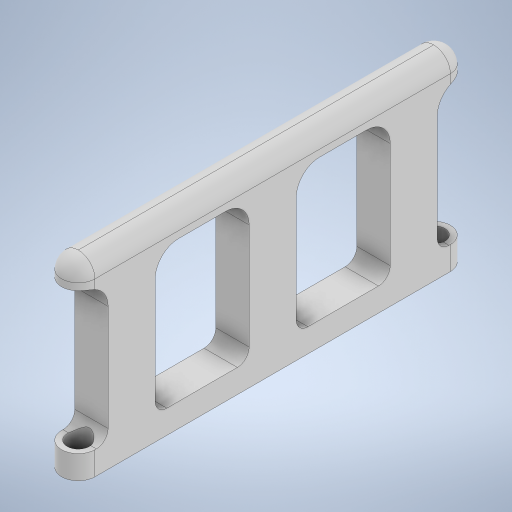
# Autodesk Inventor part: land
Saved by Autodesk Inventor 2023 (Build 270158000, 158)
## iProperties
Created: 2022-11-30
Part Number: land
Material: Generic
Document SubType Name: Modeling
Designer: user
Density: 1 g/cm^3
Appearance: Default
Author: user
Autodesk Inventor part; units mm, degrees
ref_plane "YZ Plane" through (0, 0, 0) normal (1, 0, 0) x (0, 1, 0)
ref_plane "XZ Plane" through (0, 0, 0) normal (0, 1, 0) x (-1, 0, 0)
ref_plane "XY Plane" through (0, 0, 0) normal (0, 0, 1) x (1, 0, 0)
sketch "Sketch1" plane through (0, 0, 0) normal (0, 1, 0) x (-1, 0, 0)
  circle A0 centre (0, 0) radius 4.5
  circle A1 centre (0, 0) radius 1.475
  circle A2 centre (0, 0) radius 3
  line L0 (4.5, 0) -> (4.5, -96.011)
  line L1 (-4.5, 0) -> (-4.5, -96.011)
  circle A3 centre (0, -96.011) radius 4.5
  circle A4 centre (0, -96.011) radius 1.475
  circle A5 centre (0, -96.011) radius 3
  point P0 (2.9871, -99.3766)
  point P1 (-0.7146, -91.5681)
  dimension "d0" = 9
  dimension "d1" = 2.95
  dimension "d2" = 6
  dimension "d3" = 96.011
  dimension "d5" = 9
  dimension "d6" = 2.95
  dimension "d7" = 6
  constraints: 6 centre point, 5 coincident, 4 end point, 4 point on circle, 2 tangent, 2 vertical
  measures "d0" diameter of A0
  measures "d1" diameter of A1
  measures "d2" diameter of A2
  measures "d3" distance of L0.start L0.end
  measures "d5" diameter of A3
  measures "d6" diameter of A4
  measures "d7" diameter of A5
extrude "Extrusion1" add sketch "Sketch1" along normal blind 6.35 contours A0 | L0 A3 L1 A0 | A3 | A1 | A2 | A4 | A5
sketch "Sketch2" plane through (0, 6.35, 0) normal (0, 1, 0) x (1, 0, 0)
  circle A0 centre (0, 0) radius 1.475
  dimension "d10" = 2.95
  constraints: 1 centre point, 1 coincident
  measures "d10" diameter of A0
extrude "Extrusion2" cut sketch "Sketch2" against normal blind 6.35
sketch "Sketch3" plane through (0, 6.35, 0) normal (0, 1, 0) x (1, 0, 0)
  circle A0 centre (0, 0) radius 1.475 projected
  circle A1 centre (0, 0) radius 3
  dimension "d13" = 6
  constraints: 1 centre point, 1 coincident
  measures "d13" diameter of A1
extrude "Extrusion3" cut sketch "Sketch3" against normal blind 5.08
sketch "Sketch4" plane through (0, 6.35, 0) normal (0, 1, 0) x (1, 0, 0)
  arc A0 (4.5, 96.011) -> (-4.5, 96.011) centre (0, 96.011) ccw projected
  circle A1 centre (0, 96.011) radius 1.475
  point P0 (0, 0)
  dimension "d16" = 2.95
  constraints: 1 centre point, 1 coincident
  measures "d16" diameter of A1
extrude "Extrusion4" cut sketch "Sketch4" against normal blind 6.35
sketch "Sketch5" plane through (0, 6.35, 0) normal (0, 1, 0) x (1, 0, 0)
  arc A0 (4.5, 96.011) -> (-4.5, 96.011) centre (0, 96.011) ccw projected
  circle A1 centre (0, 96.011) radius 3
  point P0 (0, 0)
  dimension "d19" = 6
  constraints: 1 centre point, 1 coincident
  measures "d19" diameter of A1
extrude "Extrusion5" cut sketch "Sketch5" against normal blind 5.08
sketch "Sketch6" plane through (0, 6.35, 0) normal (0, 1, 0) x (1, 0, 0)
  circle A0 centre (0, 0) radius 3 projected
  circle A1 centre (0, 96.011) radius 1.475 projected
  arc A2 (-4.5, 0) -> (4.5, 0) centre (0, 0) ccw projected
  line L0 (4.5, 0) -> (4.5, 96.011)
  line L1 (-4.5, 54.3555) -> (4.5, 54.3555)
  line L2 (4.5, 54.3555) -> (4.5, 41.6555)
  line L3 (4.5, 0) -> (4.5, 96.011) projected
  line L4 (4.5, 41.6555) -> (-4.5, 41.6555)
  line L5 (-4.5, 96.011) -> (-4.5, 0) projected
  line L6 (-4.5, 41.6555) -> (-4.5, 54.3555)
  dimension "d23" = 12.7
  constraints: 10 end point, 3 point on line, 1 vertical
  measures "d23" distance of L1.end L2.end
extrude "Extrusion6" add sketch "Sketch6" along normal blind 38.1 contours L5 L1 L0 L4
sketch "Sketch7" plane through (-4.5, 0, -96.011) normal (-1, 0, 0) x (0, 0, 1)
  point P0 (96.011, 0)
sketch "Sketch8" plane through (0, 6.35, 0) normal (0, 1, 0) x (1, 0, 0)
  line L0 (4.5, 41.6555) -> (-4.5, 41.6555) projected
  line L1 (0, 3.5555) -> (-4.5, 3.5555)
  line L2 (-4.5, 41.6555) -> (-4.5, 0) projected
  line L3 (-4.5, 3.5555) -> (-4.5, 16.2555)
  line L4 (-4.5, 16.2555) -> (4.5, 16.2555)
  line L5 (4.5, 0) -> (4.5, 41.6555) projected
  line L6 (4.5, 16.2555) -> (4.5, 3.5555)
  line L7 (4.5, 3.5555) -> (0, 3.5555)
  line L8 (-4.5, 54.3555) -> (4.5, 54.3555) projected
  line L9 (0, 92.4555) -> (-4.5, 92.4555)
  line L10 (-4.5, 96.011) -> (-4.5, 0) projected
  line L11 (-4.5, 92.4555) -> (-4.5, 79.7555)
  line L12 (-4.5, 79.7555) -> (4.5, 79.7555)
  line L13 (4.5, 0) -> (4.5, 96.011) projected
  line L14 (4.5, 79.7555) -> (4.5, 92.4555)
  line L15 (4.5, 92.4555) -> (0, 92.4555)
  point P0 (0, 0)
  dimension "d29" = 12.7
  constraints: 20 end point, 6 perpendicular, 6 point on line, 1 vertical
  measures "d29" distance of L9.end L11.end
extrude "Extrusion7" add sketch "Sketch8" along normal blind 38.1 contours L5 L7 L1 L2 L4 | L12 L10 L9 L15 L13
fillet "Fillet1" radius 3.175 6 edges at (0, 6.35, -3.5555) (0, 6.35, -16.2555) (0, 6.35, -41.6555) (0, 6.35, -54.3555) (0, 6.35, -79.7555) (0, 6.35, -92.4555)
sketch "Sketch9" plane through (0, 44.45, 0) normal (0, 1, 0) x (1, 0, 0)
  line L0 (-4.5, 96.011) -> (-4.5, 0) projected
  circle A0 centre (0, 0) radius 4.5
  circle A1 centre (0, 96.011) radius 1.475 projected
  circle A2 centre (0, 96.011) radius 4.5
  arc A3 (-4.5, 0) -> (4.5, 0) centre (0, 0) ccw projected
  arc A4 (4.5, 96.011) -> (-4.5, 96.011) centre (0, 96.011) ccw projected
  line L1 (-4.5, 0) -> (-4.5, 96.011)
  line L2 (4.5, 0) -> (4.5, 96.011) projected
  line L3 (4.5, 96.011) -> (4.5, 0)
  constraints: 4 end point, 4 tangent, 2 centre point, 2 coincident, 2 point on circle, 1 collinear, 1 vertical
extrude "Extrusion8" add sketch "Sketch9" along normal blind 6.35 contours A2 L2 A0 L0 | A2 | A0 | A1
fillet "Fillet2" radius 4.5 4 edges at (4.5, 50.8, -48.0055) (0, 50.8, -100.511) (-4.5, 50.8, -48.0055) (0, 50.8, 4.5)
fillet "Fillet3" radius 6.35 6 edges at (0, 44.45, -3.5555) (0, 44.45, -16.2555) (0, 44.45, -41.6555) (0, 44.45, -54.3555) (0, 44.45, -79.7555) (0, 44.45, -92.4555)
body "Solid1"
